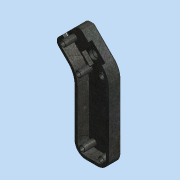
# Autodesk Inventor part: CaseRight
Saved by Autodesk Inventor 2015 (Build 190159000, 159)
## iProperties
Created: 2015-11-11
Part Number: CaseRight
Material: ABS Plastic
Document SubType Name: Modeling
Designer: Raphael
Density: 1.06 g/cm^3
Appearance: Plate
wheel_diameter: 1.000 in
Author: Raphael
Autodesk Inventor part; units mm, degrees
ref_plane "YZ Plane" through (0, 0, 0) normal (1, 0, 0) x (0, 1, 0)
sketch "Sketch1" plane through (0, 0, 0) normal (0, 0, 1) x (1, 0, 0)
  line L0 (0, -10.521024) -> (0, -63.5)
  line L1 (12.7, -76.2) -> (25.4, -76.2)
  line L2 (38.1, -63.5) -> (38.1, 5.260512)
  line L3 (30.660512, 23.221024) -> (8.980256, 44.901281)
  line L4 (0, 44.901281) -> (-17.960512, 26.940768)
  line L5 (-17.960512, 17.960512) -> (-7.439488, 7.439488)
  line L6 (-38.626051, 0) -> (53.956308, 0)
  arc A0 (38.1, 5.260512) -> (30.660512, 23.221024) centre (12.7, 5.260512) ccw
  arc A1 (0, -10.521024) -> (-7.439488, 7.439488) centre (-25.4, -10.521024) ccw
  arc A2 (-17.960512, 26.940768) -> (-17.960512, 17.960512) centre (-13.470384, 22.45064) ccw
  arc A3 (8.980256, 44.901281) -> (0, 44.901281) centre (4.490128, 40.411153) ccw
  arc A4 (0, -63.5) -> (12.7, -76.2) centre (12.7, -63.5) ccw
  arc A5 (25.4, -76.2) -> (38.1, -63.5) centre (25.4, -63.5) ccw
  point P0 (0, 0)
  point P1 (0, -76.2)
  point P2 (-22.45064, 22.45064)
  dimension "d0" = 45
  dimension "d1" = 38.1
  dimension "d2" = 38.1
  dimension "d3" = 76.2
  dimension "d4" = 31.75
  dimension "d5" = 25.4
  dimension "d6" = 6.35
  dimension "d7" = 12.7
  constraints: 12 end point, 12 point on circle, 12 tangent, 6 centre point, 6 point on line, 3 equal radius, 2 perpendicular, 1 parallel, 1 vertical
  measures "d0" angle of L6 L5
  measures "d1" distance between parallel lines of L2 L0
  measures "d2" distance between parallel lines of L3 L5
  measures "d3" distance of point (0, 0) point (0, -76.2)
  measures "d4" distance of point (-22.451, 22.451) point (0, 0)
  measures "d5" radius of A0
  measures "d6" radius of A2
  measures "d7" radius of A4
extrude "Extrusion1" add sketch "Sketch1" against normal blind 15.875
shell "Shell1" thickness 3.175 removed faces 1 at (25.4, -22.920171, 0)
sketch "Sketch2" plane through (30.660512, 23.221024, -15.875) normal (0.7071068, 0.7071068, 0) x (-0.7071068, 0.7071068, 0)
  line L0 (0, 15.875) -> (30.660513, 15.875)
  line L1 (0, 15.875) -> (0, 0)
  line L2 (30.660513, 0) -> (0, 0)
  line L3 (30.660513, 15.875) -> (30.660513, 0)
  line L4 (30.660513, 15.875) -> (15.781537, 15.875)
  line L5 (20.6375, 15.875) -> (1.5875, 15.875)
  line L6 (1.5875, 15.875) -> (1.5875, 11.90625)
  line L7 (1.5875, 11.90625) -> (20.6375, 11.90625)
  line L8 (20.6375, 11.90625) -> (20.6375, 15.875)
  point P0 (5.260512, 15.875)
  point P1 (15.330256, 0)
  point P2 (11.1125, 11.90625)
  dimension "d11" = 19.05
  dimension "d12" = 3.96875
  dimension "d53" = 1.5875
  constraints: 8 end point, 2 midpoint, 2 parallel, 1 horizontal, 1 perpendicular, 1 point on line
  measures "d11" distance between parallel lines of L8 L6
  measures "d12" distance between parallel lines of L0 L7
  measures "d53" distance between parallel lines of L1 L6
extrude "Extrusion2" cut sketch "Sketch2" against normal up to next contours L0 L8 L7 L6
sketch "Sketch3" plane through (29.53798, 24.343556, -3.96875) normal (0, 0, 1) x (0.7071068, 0.7071068, 0)
  line L0 (-3.175, 0) -> (-3.175, 19.05)
  line L1 (0, 0) -> (-3.175, 0)
  line L2 (0, 19.05) -> (0, 0)
  line L3 (0, 19.05) -> (-3.175, 19.05)
  line L4 (-3.175, 16.66875) -> (-8.40026, 16.66875)
  line L5 (-8.40026, 2.38125) -> (-3.175, 2.38125)
  line L6 (0, 0) -> (-3.175, 0)
  arc A0 (-8.40026, 16.66875) -> (-8.40026, 2.38125) centre (-8.40026, 9.525) ccw construction
  line L7 (-3.175, 0) -> (-3.175, 19.05)
  circle A1 centre (-8.40026, 9.525) radius 12.7 construction
  circle A2 centre (-8.40026, 9.525) radius 13.49375
  circle A3 centre (-8.40026, 9.525) radius 4.7625
  line L8 (-8.40026, 16.66875) -> (-21.10026, 16.66875)
  line L9 (-21.10026, 16.66875) -> (-21.10026, 2.38125)
  line L10 (-21.10026, 2.38125) -> (-8.40026, 2.38125)
  line L11 (-20.30651, 15.875) -> (-13.95651, 15.875)
  line L12 (-13.95651, 15.875) -> (-13.95651, 3.175)
  line L13 (-13.95651, 3.175) -> (-20.30651, 3.175)
  line L14 (-20.30651, 3.175) -> (-20.30651, 15.875)
  line L15 (-13.16276, 16.66875) -> (-13.16276, 2.38125) construction
  line L16 (-3.175, 2.38125) -> (-3.175, 16.66875)
  line L17 (-3.175, 29.073013) -> (-3.175, -1.5875)
  line L18 (0, 19.05) -> (0, 0)
  point P0 (-38.1, 3.673012)
  point P1 (-3.175, 9.525)
  point P2 (-20.30651, 9.525)
  point P3 (-21.10026, 9.525)
  point P4 (-3.175, 9.525)
  point P5 (0, 9.525)
  point P6 (-3.175, 9.525)
  point P7 (0, 9.525)
  dimension "d15" = 25.4
  dimension "d16" = 26.9875
  dimension "d21" = 9.525
  dimension "d23" = 0.79375
  dimension "d24" = 0.79375
  dimension "d25" = 0.79375
  dimension "d48" = 6.35
  dimension "d49" = 12.7
  constraints: 22 end point, 8 midpoint, 4 horizontal alignment, 4 perpendicular, 3 centre point, 3 coincident, 3 horizontal, 3 parallel, 3 tangent, 2 point on circle, 2 point on line, 1 collinear, 1 vertical alignment, 3 other
  measures "d16" diameter of A2
  measures "d21" diameter of A3
  measures "d23" distance between parallel lines of L9 L14
  measures "d24" distance between parallel lines of L10 L13
  measures "d25" distance between parallel lines of L15 L12
  measures "d48" distance of L11.start L11.end
  measures "d49" distance of L13.end L11.start
extrude "Extrusion3" cut sketch "Sketch3" along normal through all contours L1 L2 L3 L17 A2 L10 L5 L0 | L4 L8 A2 L17 L0 | A2 L9
extrude "Extrusion4" add sketch "Sketch3" against normal up to surface (8.73125 mm away) separate body contours L5 L10 A2 L13 L12 L11 L8 L4 L0 | L10 L9 A2 | A2 L9 L8 | A2 L9 L14
sketch "Sketch4" plane through (12.7, -73.025, -12.7) normal (0, 0, 1) x (1, 0, 0)
  circle A0 centre (4.162907, 98.163867) radius 4.7625
  circle A1 centre (4.162907, 98.163867) radius 3.96875
  point P0 (-12.7, 73.025)
  dimension "d26" = 0.79375
  constraints: 1 centre point, 1 coincident
  measures "d26" radial gap between concentric circles of A0 A1
ref_plane "Work Plane1" through (29.53798, 24.343556, -7.14375) normal (0, 0, 1) x (0.7071068, -0.7071068, 0)
extrude "Extrusion5" add sketch "Sketch4" along normal up to surface (5.55625 mm away) bodies 2
sketch "Sketch5" plane through (12.7, -73.025, -12.7) normal (0, 0, 1) x (1, 0, 0)
  line L0 (-5.964808, 115.681217) -> (15.715448, 94.00096)
  arc A0 (-5.964808, 115.681217) -> (-10.454936, 115.681217) centre (-8.209872, 113.436153) ccw
  line L1 (-28.415448, 97.720704) -> (-10.454936, 115.681217)
  arc A1 (-28.415448, 97.720704) -> (-28.415448, 93.230576) centre (-26.170384, 95.47564) ccw
  line L2 (-17.894424, 82.709552) -> (-28.415448, 93.230576)
  arc A2 (-9.525, 62.503976) -> (-17.894424, 82.709552) centre (-38.1, 62.503976) ccw
  line L3 (-9.525, 9.525) -> (-9.525, 62.503976)
  arc A3 (-9.525, 9.525) -> (0, 0) centre (0, 9.525) ccw
  line L4 (12.7, 0) -> (0, 0)
  arc A4 (12.7, 0) -> (22.225, 9.525) centre (12.7, 9.525) ccw
  line L5 (22.225, 78.285512) -> (22.225, 9.525)
  arc A5 (22.225, 78.285512) -> (15.715448, 94.00096) centre (0, 78.285512) ccw
  circle A6 centre (-4.368895, 5.156105) radius 3.34645
  circle A7 centre (-4.368895, 5.156105) radius 2.5527
  arc A8 (-9.525, 9.525) -> (0, 0) centre (0, 9.525) ccw
  line L6 (-4.368895, 5.156105) -> (0, 9.525) construction
  line L7 (12.7, 0) -> (0, 0)
  line L8 (6.35, 0) -> (6.35, 62.503976) construction
  circle A9 centre (17.068895, 5.156105) radius 3.34645
  circle A10 centre (17.068895, 5.156105) radius 2.5527
  circle A11 centre (-8.608426, 74.719786) radius 3.34645
  circle A12 centre (-8.608426, 74.719786) radius 2.5527
  circle A13 centre (17.441506, 85.510021) radius 3.34645
  circle A14 centre (17.441506, 85.510021) radius 2.5527
  arc A15 (-9.525, 62.503976) -> (-17.894424, 82.709552) centre (-38.1, 62.503976) ccw
  arc A16 (22.225, 78.285512) -> (15.715448, 94.00096) centre (0, 78.285512) ccw
  arc A17 (22.225, 78.285512) -> (15.715448, 94.00096) centre (0, 78.285512) ccw
  line L9 (-38.1, 62.503976) -> (0, 78.285512) construction
  line L10 (17.441506, 85.510021) -> (-8.608426, 74.719786) construction
  circle A18 centre (-25.927917, 95.47564) radius 3.34645
  circle A19 centre (-25.927917, 95.47564) radius 2.5527
  line L11 (-28.415448, 97.720704) -> (-10.454936, 115.681217)
  line L12 (-17.894424, 82.709552) -> (-28.415448, 93.230576)
  line L13 (15.715448, 94.00096) -> (-5.964808, 115.681217)
  point P0 (-12.7, 73.025)
  point P1 (14.894501, 94.821908)
  point P2 (-0.939376, 110.655785)
  dimension "d30" = 6.6929
  dimension "d31" = 5.1054
  dimension "d32" = 45
  dimension "d33" = 6.6929
  dimension "d34" = 5.1054
  dimension "d35" = 6.6929
  dimension "d36" = 5.1054
  dimension "d41" = 6.6929
  dimension "d42" = 5.1054
  constraints: 10 centre point, 8 end point, 5 coincident, 5 tangent, 2 symmetric about line, 1 collinear, 1 midpoint, 1 vertical, 2 other
  measures "d30" diameter of A6
  measures "d31" diameter of A7
  measures "d32" angle of L4 L6
  measures "d33" diameter of A11
  measures "d34" diameter of A12
  measures "d35" diameter of A13
  measures "d36" diameter of A14
  measures "d41" diameter of A18
  measures "d42" diameter of A19
extrude "Extrusion6" add sketch "Sketch5" along normal up to surface (12.7 mm away) contours A13 | A11 | A6 | A9 | A18 bodies 1
extrude "Extrusion7" cut sketch "Sketch5" against normal through all contours A7 | A10 | A12 | A14 | A19 bodies 1
chamfer "Chamfer1" distance 3.175 angle 45 12 edges at (36.1665, 14.9807, -15.875) (38.1, -29.1197, -15.875) (34.3803, -72.4803, -15.875) (19.05, -76.2, -15.875) (3.7197, -72.4803, -15.875) (0, -37.0105, -15.875) (-1.9335, -0.8009, -15.875) (-12.7, 12.7, -15.875) (-19.8204, 22.4506, -15.875) (-8.9803, 35.921, -15.875) (4.4901, 46.7612, -15.875) (19.8204, 34.0612, -15.875)
sketch "Sketch6" plane through (12.7, -73.025, -12.7) normal (0, 0, 1) x (1, 0, 0)
  line L0 (-4.256083, 98.725133) -> (4.724173, 89.744877)
  line L1 (-8.746211, 94.235005) -> (-4.256083, 98.725133)
  line L2 (0.234045, 85.254749) -> (-8.746211, 94.235005)
  line L3 (4.724173, 89.744877) -> (0.234045, 85.254749)
  point P0 (-12.7, 73.025)
ref_plane "Work Plane2" through (29.53798, 24.343556, -10.31875) normal (0, 0, 1) x (0.7071068, -0.7071068, 0)
extrude "Extrusion8" add sketch "Sketch6" along normal up to surface (2.38125 mm away) bodies 2
sketch "Sketch7" plane through (-17.960512, 26.940768, -12.7) normal (-0.7071068, 0.7071068, 0) x (0, 0, 1)
  line L0 (0, 0) -> (0, 25.4) projected
  line L1 (12.7, 0) -> (0, 0) projected
  line L2 (12.7, 25.4) -> (12.7, 0) projected
  line L3 (12.7, 25.4) -> (0, 25.4) projected
  line L4 (12.7, 19.05) -> (7.9375, 19.05)
  line L5 (7.9375, 19.05) -> (7.9375, 6.35)
  line L6 (7.9375, 6.35) -> (12.7, 6.35)
  line L7 (12.7, 6.35) -> (12.7, 19.05)
  point P0 (12.7, -6.35)
  point P1 (7.9375, 12.7)
  point P2 (0, 12.7)
  dimension "d54" = 12.7
  dimension "d55" = 4.7625
  constraints: 8 end point, 2 midpoint, 2 parallel, 1 horizontal, 1 horizontal alignment, 1 perpendicular, 1 point on line
  measures "d54" distance of L4.end L5.end
  measures "d55" distance of L5.end L6.end
extrude "Extrusion9" cut sketch "Sketch7" against normal up to surface (3.175 mm away) contours L6 L5 L4 L2 bodies 1
fillet "Fillet1" radius 1.5875 2 edges at (-3.3676, 39.2886, -4.7625) (-12.3479, 30.3084, -4.7625)
equation "\"d15\" = wheel_diameter"
equation "\"wheel_diameter\" = 25.4"
body "Solid1"
body "Solid2"
